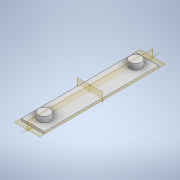
# Autodesk Inventor part: Tile_Cover
Saved by Autodesk Inventor 2022.4 (Build 264492010, 492A)
## iProperties
Created: 2025-02-20
Part Number: Tile_Cover
Material: Generic
Document SubType Name: Modeling
Designer: jan-m
Density: 1 g/cm^3
Appearance: Default
Author: jan-m
Autodesk Inventor part; units mm, degrees
sketch "Sketch1" plane through (0, 0, 0) normal (0, 1, 0) x (-1, 0, 0)
  line L0 (5, -25) -> (-5, -25)
  line L1 (-5, -25) -> (-5, 25)
  line L2 (-5, 25) -> (5, 25)
  line L3 (5, 25) -> (5, -25)
  line L4 (0, -34.825) -> (0, 34.825) projected
  line L5 (-7, 0) -> (7, 0) projected
  point P0 (0, 0)
  point P1 (0, -25)
  point P2 (5, 0)
  dimension "d0" = 10
  dimension "d1" = 50
  constraints: 8 end point, 2 midpoint, 2 parallel, 2 point on line, 1 horizontal, 1 perpendicular
  measures "d0" distance of L0.start L0.end
  measures "d1" distance of L2.end L0.start
extrude "Extrusion1" add sketch "Sketch1" along normal mid plane 1
sketch "Sketch2" plane through (0, 0.5, 0) normal (0, 1, 0) x (1, 0, 0)
  circle A0 centre (0, 20) radius 2.5
  line L0 (5, 25) -> (-5, 25) projected
  line L1 (-5, 25) -> (-5, -25) projected
  circle A1 centre (0, -20) radius 2.5
  point P0 (0, 0)
  dimension "d4" = 5
  dimension "d5" = 5
  dimension "d6" = 5
  dimension "d9" = 360
  constraints: 2 centre point, 5 other
  measures "d4" diameter of A0
  measures "d5" distance from line of L0 A0.centre
  measures "d6" distance from line of L1 A0.centre
extrude "Extrusion2" add sketch "Sketch2" along normal blind 2.5
body "Solid1"
